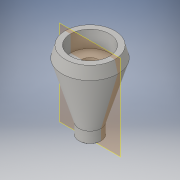
# Autodesk Inventor part: Caufield_Stack
Saved by Autodesk Inventor 2016 (Build 200138000, 138)
## iProperties
Created: 2018-01-09
Part Number: Caufield_Stack
Material: Generic
Document SubType Name: Modeling
Designer: caufield58738
Density: 1 g/cm^3
Appearance: Default
Author: caufield58738
Autodesk Inventor part; units mm, degrees
ref_plane "YZ Plane" through (0, 0, 0) normal (1, 0, 0) x (0, 1, 0)
ref_plane "XZ Plane" through (0, 0, 0) normal (0, 1, 0) x (-1, 0, 0)
sketch "Stack Sketch" plane through (0, 0, 0) normal (0, 0, 1) x (1, 0, 0)
  line L0 (0, 0) -> (6.35, 0)
  line L1 (6.35, 0) -> (6.35, 6.35)
  line L2 (6.35, 6.35) -> (15.875, 38.1)
  line L3 (0, 44.45) -> (0, 0)
  line L4 (15.875, 38.1) -> (15.875, 46.0795) construction
  line L5 (15.875, 38.1) -> (14.1735, 44.45)
  line L6 (14.1735, 44.45) -> (0, 44.45)
  dimension "d0" = 6.35
  dimension "d1" = 38.1
  dimension "d5" = 6.35
  dimension "d6" = 44.45
  dimension "d7" = 15
  dimension "d17" = 15.875
  constraints: 14 end point, 2 horizontal, 2 perpendicular, 1 vertical
  measures "d0" distance of L0.end L1.end
  measures "d1" distance from line of L0 L2.end
  measures "d5" distance of L0.start L0.end
  measures "d6" distance of L3.start L0.start
  measures "d7" angle of L4 L5
  measures "d17" distance from line of L3 L2.end
revolve "Stack Revolve" add sketch "Stack Sketch" angle 360 about axis through (0, 44.45, 0) along (0, -1, 0)
sketch "Stack Hole Sketch" plane through (0, 44.45, 0) normal (0, 1, 0) x (1, 0, 0)
  point P0 (0, 0)
  point P1 (0, 0)
  constraints: 1 coincident
hole "Stack Hole" at (0, 44.45, 0) direction (0, -1, 0) diameter 9.525 depth 38.1 counterbore diameter 22.225 counterbore depth 9.525
chamfer "Bottom Chamfer" distance 0.254 angle 45 1 edges at (-6.35, 0, 0)
body "Solid1"
